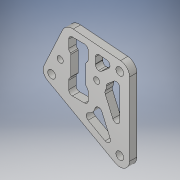
# Autodesk Inventor part: 前後機構_下側板
Saved by Autodesk Inventor 2019.4 (Build 234330000, 330)
## iProperties
Created: 2021-12-05
Part Number: 前後機構_下側板
Material: アルミニウム 6061
Document SubType Name: Modeling
Designer: 堀川皓史
Density: 2.7 g/cm^3
Appearance: アルミニウム - フラット
Author: 堀川皓史
Autodesk Inventor part; units mm, degrees
ref_plane "YZ Plane" through (0, 0, 0) normal (1, 0, 0) x (0, 1, 0)
ref_plane "XZ Plane" through (0, 0, 0) normal (0, 1, 0) x (-1, 0, 0)
ref_plane "XY Plane" through (0, 0, 0) normal (0, 0, 1) x (1, 0, 0)
sketch "スケッチ1" plane through (0, 0, 0) normal (0, 0, 1) x (1, 0, 0)
  line L0 (-7.5, 32.0148) -> (7.5, 32.0148) construction
  line L1 (7.5, 32.0148) -> (7.5, -42.6706) construction
  line L2 (7.5, -42.6706) -> (-7.5, -42.6706) construction
  line L3 (-7.5, -42.6706) -> (-7.5, 32.0148) construction
  arc A0 (-12.7011, -3.0588) -> (-14.1768, 1.4689) centre (-11, 0) ccw construction
  circle A1 centre (17, 15) radius 9.5 construction
  circle A2 centre (17, -15) radius 9.5 construction
  circle A3 centre (-11, 0) radius 1.6
  line L4 (-11, 0) -> (17, 15) construction
  line L5 (17, 15) -> (17, -15) construction
  line L6 (17, -15) -> (-11, 0) construction
  circle A4 centre (17, 15) radius 1.6
  circle A5 centre (17, -15) radius 1.6
  line L7 (3, -2.5) -> (-3, -2.5) construction
  line L8 (-2.5, -3.5) -> (2.5, -3.5)
  arc A6 (2.5, -3.5) -> (4, -2) centre (2.5, -2) ccw
  line L9 (-4, 1.3297) -> (-4, -2)
  arc A7 (-4, -2) -> (-2.5, -3.5) centre (-2.5, -2) ccw
  line L10 (2.5, 17.5) -> (-2.5, 17.5)
  arc A8 (4, 16) -> (2.5, 17.5) centre (2.5, 16) ccw
  line L11 (-3, 16.5) -> (3, 16.5) construction
  arc A9 (3.1, 3) -> (3.325, 2.5824) centre (3.6, 3) ccw
  line L12 (3.1, 11) -> (3.1, 3)
  arc A10 (4, 1.3297) -> (3.325, 2.5824) centre (2.5, 1.3297) ccw
  line L13 (4, -2) -> (4, 1.3297)
  line L14 (-3, -2.5) -> (-3, 16.5) construction
  line L15 (3, 16.5) -> (3, -2.5) construction
  arc A11 (-3.325, 2.5824) -> (-4, 1.3297) centre (-2.5, 1.3297) ccw
  arc A12 (-3.325, 2.5824) -> (-3.1, 3) centre (-3.6, 3) ccw
  line L16 (4, 12.6703) -> (4, 16)
  arc A13 (3.325, 11.4176) -> (4, 12.6703) centre (2.5, 12.6703) ccw
  arc A14 (3.325, 11.4176) -> (3.1, 11) centre (3.6, 11) ccw
  arc A15 (-2.5, 17.5) -> (-4, 16) centre (-2.5, 16) ccw
  line L17 (-4, 16) -> (-4, 12.6703)
  arc A16 (-4, 12.6703) -> (-3.325, 11.4176) centre (-2.5, 12.6703) ccw
  arc A17 (-3.1, 11) -> (-3.325, 11.4176) centre (-3.6, 11) ccw
  line L18 (-3.1, 11) -> (-3.1, 3)
  circle A18 centre (-7.5, 7) radius 1.25
  circle A19 centre (7.5, 7) radius 1.25
  arc A20 (21, 15) -> (17.3071, 18.9882) centre (17, 15) ccw
  arc A21 (15.0558, -18.4958) -> (21, -15) centre (17, -15) ccw
  arc A22 (-2.1545, 20.4867) -> (-6.5845, 17.8886) centre (-2.5, 16) ccw
  line L19 (-6.5845, 17.8886) -> (-14.1768, 1.4689)
  line L20 (-2.1545, 20.4867) -> (17.3071, 18.9882)
  line L21 (21, 15) -> (21, -15)
  line L22 (15.0558, -18.4958) -> (-12.7011, -3.0588)
  arc A23 (-14.1768, 1.4689) -> (-12.7011, -3.0588) centre (-11, 0) ccw
  point P0 (0, 0)
  point P1 (0, 7)
  point P2 (11.1864, 31.6552)
  dimension "d0" = 15
  dimension "d1" = 7.5
  dimension "d2" = 7
  dimension "d3" = 19
  dimension "d4" = 19
  dimension "d5" = 3.2
  dimension "d6" = 30
  dimension "d7" = 3.2
  dimension "d8" = 3.2
  dimension "d9" = 6
  dimension "d10" = 19
  dimension "d11" = 3
  dimension "d12" = 9.5
  dimension "d13" = 1
  dimension "d14" = 8
  dimension "d15" = 4
  dimension "d16" = 0.1
  dimension "d17" = 0.1
  dimension "d18" = 1
  dimension "d19" = 1
  dimension "d20" = 1
  dimension "d21" = 1.5
  dimension "d22" = 1
  dimension "d23" = 1.5
  dimension "d24" = 0.5
  dimension "d25" = 1
  dimension "d26" = 1.5
  dimension "d27" = 0.5
  dimension "d28" = 1.5
  dimension "d29" = 0.5
  dimension "d30" = 0.5
  dimension "d31" = 1.5
  dimension "d32" = 2.5
  dimension "d33" = 2.5
  dimension "d34" = 15
  dimension "d35" = 7.5
  dimension "d38" = 7
  dimension "d39" = 4
  dimension "d40" = 4
  dimension "d41" = 3
  constraints: 46 end point, 34 point on circle, 29 tangent, 24 centre point, 7 horizontal alignment, 7 parallel, 6 coincident, 4 perpendicular, 4 vertical, 3 equal radius, 2 horizontal, 1 equal length, 1 vertical alignment
  measures "d0" distance between parallel lines of L1 L3
  measures "d1" distance from line of point (0, 0) L3
  measures "d2" diameter of A0
  measures "d3" diameter of A1
  measures "d4" diameter of A2
  measures "d5" diameter of A3
  measures "d6" distance of L4.end L5.end
  measures "d7" diameter of A4
  measures "d8" diameter of A5
  measures "d9" distance of L11.start L11.end
  measures "d10" distance of L11.end L7.start
  measures "d11" distance from line of point (0, 7) L14
  measures "d12" distance from line of point (0, 7) L11
  measures "d13" distance between parallel lines of L7 L8
  measures "d14" distance of L18.start L18.end
  measures "d15" vertical distance of point (0, 7) L18.end
  measures "d16" distance between parallel lines of L18 L14
  measures "d17" distance between parallel lines of L15 L12
  measures "d18" distance between parallel lines of L14 L9
  measures "d19" distance between parallel lines of L15 L13
  measures "d20" distance between parallel lines of L11 L10
  measures "d21" radius of A15
  measures "d22" distance between parallel lines of L14 L17
  measures "d23" radius of A16
  measures "d24" radius of A17
  measures "d25" distance between parallel lines of L15 L16
  measures "d26" radius of A13
  measures "d27" radius of A14
  measures "d28" radius of A11
  measures "d29" radius of A12
  measures "d30" radius of A9
  measures "d31" radius of A10
  measures "d32" diameter of A18
  measures "d33" diameter of A19
  measures "d34" distance of A19.centre A18.centre
  measures "d35" distance of point (0, 7) A18.centre
  measures "d38" distance of point (0, 0) point (0, 7)
  measures "d39" radius of A20
  measures "d40" radius of A21
  measures "d41" radial gap between concentric circles of A15 A22
extrude "押し出し1" add sketch "スケッチ1" along normal blind 3
sketch "スケッチ2" plane through (0, 0, 3) normal (0, 0, 1) x (1, 0, 0)
  circle A0 centre (17, -15) radius 1.6 projected
  circle A1 centre (7.5, 7) radius 1.25 projected
  line L0 (17, -15) -> (7.5, 7) construction
  line L1 (4, 1.3297) -> (4, -2) projected
  arc A2 (2.5, -3.5) -> (4, -2) centre (2.5, -2) ccw projected
  line L2 (2.5, -3.5) -> (-2.5, -3.5) projected
  line L3 (7, 3.1129) -> (7, -2)
  arc A3 (2.5, -6.5) -> (7, -2) centre (2.5, -2) ccw
  line L4 (2.5, -6.5) -> (-0.3412, -6.5)
  arc A4 (13.7906, -12.6126) -> (13.1292, -13.9915) centre (17, -15) ccw
  line L5 (7, 3.1129) -> (13.7906, -12.6126)
  line L6 (13.1292, -13.9915) -> (-0.3412, -6.5)
  line L7 (-12.7011, -3.0588) -> (15.0558, -18.4958) projected
  circle A5 centre (17, 15) radius 1.6 projected
  line L8 (7.5, 7) -> (17, 15) construction
  arc A6 (15.6385, 11.2388) -> (17, 11) centre (17, 15) ccw
  arc A7 (10.7094, 4.6126) -> (11.438, 7.7015) centre (7.5, 7) ccw
  line L9 (11.438, 7.7015) -> (15.6385, 11.2388)
  line L10 (17, 11) -> (17, -9.955)
  line L11 (17, -9.955) -> (10.7094, 4.6126)
  line L12 (21, -15) -> (21, 15) projected
  arc A8 (3.325, 11.4176) -> (4, 12.6703) centre (2.5, 12.6703) ccw projected
  line L13 (4, 16) -> (4, 12.6703) projected
  arc A9 (4, 16) -> (2.5, 17.5) centre (2.5, 16) ccw projected
  arc A10 (6.6399, 10.9064) -> (7, 12.6703) centre (2.5, 12.6703) ccw
  line L14 (7, 12.6703) -> (7, 16)
  arc A11 (7, 16) -> (6.9322, 16.7782) centre (2.5, 16) ccw
  arc A12 (8.8615, 10.7612) -> (6.6399, 10.9064) centre (7.5, 7) ccw
  arc A13 (13.2152, 16.2944) -> (13.062, 14.2985) centre (17, 15) ccw
  line L15 (6.9322, 16.7782) -> (13.2152, 16.2944)
  line L16 (13.062, 14.2985) -> (8.8615, 10.7612)
  line L17 (17.3071, 18.9882) -> (-2.1545, 20.4867) projected
  point P0 (0, 0)
  dimension "d44" = 3
  dimension "d45" = 4
  dimension "d46" = 2
  dimension "d47" = 3
  dimension "d48" = 4
  dimension "d49" = 4
  dimension "d51" = 4
  dimension "d52" = 2
  dimension "d53" = 2
  dimension "d54" = 3
  dimension "d55" = 4
  dimension "d56" = 4
  dimension "d57" = 2
  dimension "d58" = 3
  constraints: 24 end point, 16 point on circle, 8 centre point, 7 parallel, 5 coincident, 4 other
  measures "d44" radial gap between concentric circles of A2 A3
  measures "d45" radius of A4
  measures "d46" distance between parallel lines of L0 L5
  measures "d47" distance between parallel lines of L7 L6
  measures "d48" radius of A7
  measures "d49" radius of A6
  measures "d51" distance between parallel lines of L12 L10
  measures "d52" distance between parallel lines of L0 L11
  measures "d53" distance between parallel lines of L9 L8
  measures "d54" distance between parallel lines of L13 L14
  measures "d55" radius of A12
  measures "d56" radius of A13
  measures "d57" distance between parallel lines of L8 L16
  measures "d58" distance between parallel lines of L17 L15
extrude "押し出し2" cut sketch "スケッチ2" against normal blind 3 contours L5 A4 L6 L4 A3 L3 | A6 L10 L11 A7 L9 | A10 L14 A11 L15 A13 L16 A12
fillet "フィレット1" radius 1.5 14 edges at (6.9322, 16.7782, 1.5) (6.6399, 10.9064, 1.5) (8.8615, 10.7612, 1.5) (13.062, 14.2985, 1.5) (13.2152, 16.2944, 1.5) (15.6385, 11.2388, 1.5) (17, 11, 1.5) (11.438, 7.7015, 1.5) (10.7094, 4.6126, 1.5) (17, -9.955, 1.5) (-0.3412, -6.5, 1.5) (13.7906, -12.6126, 1.5) (13.1292, -13.9915, 1.5) (7, 3.1129, 1.5)
fillet_without_effect "フィレット2"
equation "\"d1\" = 0.5 * d0"
equation "\"d12\" = 0.5 * d10"
